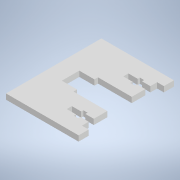
# Autodesk Inventor part: Soporte_Plug_Alimentacion
Saved by Autodesk Inventor 2020.1 (Build 241239000, 239)
## iProperties
Created: 2019-12-12
Part Number: Soporte_Plug_Alimentacion
Material: Generic
Document SubType Name: Modeling
Designer: Daniel
Density: 1 g/cm^3
Appearance: Default
Author: Daniel
Autodesk Inventor part; units mm, degrees
ref_plane "YZ Plane" through (0, 0, 0) normal (1, 0, 0) x (0, 1, 0)
ref_plane "XZ Plane" through (0, 0, 0) normal (0, 1, 0) x (-1, 0, 0)
ref_plane "XY Plane" through (0, 0, 0) normal (0, 0, 1) x (1, 0, 0)
sketch "Sketch1" plane through (0, 0, 0) normal (0, 1, 0) x (-1, 0, 0)
  line L0 (38.3151, 0) -> (38.3151, -28.25)
  line L1 (38.3151, -28.25) -> (-4.6849, -28.25)
  line L2 (-4.6849, -28.25) -> (-4.6849, -22.25)
  line L3 (-4.6849, -22.25) -> (-0.6849, -22.25)
  line L4 (-0.6849, -22.25) -> (-0.6849, -18.25)
  line L5 (-0.6849, -18.25) -> (4.3151, -18.25)
  line L6 (4.3151, -18.25) -> (4.3151, -19.525)
  line L7 (4.3151, -19.525) -> (6.8151, -19.525)
  line L8 (6.8151, -13.975) -> (4.3151, -13.975)
  line L9 (4.3151, -13.975) -> (4.3151, -15.25)
  line L10 (4.3151, -15.25) -> (-0.6849, -15.25)
  line L11 (-0.6849, -15.25) -> (-0.6849, -7.25)
  line L12 (-0.6849, -7.25) -> (19.3151, -7.25)
  line L13 (19.3151, -7.25) -> (19.3151, -5.15)
  line L14 (19.3151, -5.15) -> (28.3151, -5.15)
  line L15 (28.3151, -5.15) -> (28.3151, 0)
  line L16 (0, 0) -> (38.3151, 0) construction
  line L17 (6.8151, -15.25) -> (12.3151, -15.25)
  line L18 (12.3151, -15.25) -> (12.3151, -18.25)
  line L19 (12.3151, -18.25) -> (6.8151, -18.25)
  line L20 (6.8151, -19.525) -> (6.8151, -18.25)
  line L21 (6.8151, -15.25) -> (6.8151, -13.975)
  line L22 (38.3151, 0) -> (38.3151, 28.25)
  line L23 (38.3151, 28.25) -> (-4.6849, 28.25)
  line L24 (-4.6849, 28.25) -> (-4.6849, 22.25)
  line L25 (-4.6849, 22.25) -> (-0.6849, 22.25)
  line L26 (-0.6849, 22.25) -> (-0.6849, 18.25)
  line L27 (-0.6849, 18.25) -> (4.3151, 18.25)
  line L28 (4.3151, 18.25) -> (4.3151, 19.525)
  line L29 (4.3151, 19.525) -> (6.8151, 19.525)
  line L30 (6.8151, 13.975) -> (4.3151, 13.975)
  line L31 (4.3151, 13.975) -> (4.3151, 15.25)
  line L32 (4.3151, 15.25) -> (-0.6849, 15.25)
  line L33 (-0.6849, 15.25) -> (-0.6849, 7.25)
  line L34 (-0.6849, 7.25) -> (19.3151, 7.25)
  line L35 (19.3151, 7.25) -> (19.3151, 5.15)
  line L36 (19.3151, 5.15) -> (28.3151, 5.15)
  line L37 (28.3151, 5.15) -> (28.3151, 0)
  line L38 (6.8151, 15.25) -> (12.3151, 15.25)
  line L39 (12.3151, 15.25) -> (12.3151, 18.25)
  line L40 (12.3151, 18.25) -> (6.8151, 18.25)
  line L41 (6.8151, 19.525) -> (6.8151, 18.25)
  line L42 (6.8151, 15.25) -> (6.8151, 13.975)
  dimension "d0" = 5.55
  dimension "d1" = 2.5
  dimension "d2" = 3
  dimension "d3" = 6
  dimension "d4" = 5
  dimension "d7" = 4
  dimension "d9" = 24
  dimension "d10" = 17
  dimension "d11" = 10.3
  dimension "d12" = 9
  dimension "d13" = 14.5
  dimension "d14" = 8
  dimension "d15" = 4
  dimension "d16" = 10
  constraints: 86 end point, 20 symmetric about line, 18 perpendicular, 9 point on line, 4 collinear, 3 horizontal, 2 parallel, 1 other
  measures "d0" distance of L7.end L8.start
  measures "d1" distance of L6.end L7.end
  measures "d2" distance between parallel lines of L10 L5
  measures "d3" distance of L1.end L2.end
  measures "d4" distance of L4.end L5.end
  measures "d7" distance of L2.end L3.end
  measures "d9" distance between parallel lines of L2 L13
  measures "d10" distance between parallel lines of L2 L18
  measures "d11" diameter of L14 L16
  measures "d12" distance of L13.end L14.end
  measures "d13" diameter of L12 L16
  measures "d14" distance of L10.end L11.end
  measures "d15" distance of L3.end L4.end
  measures "d16" distance between parallel lines of L0 L15
extrude "Extrusion1" add sketch "Sketch1" along normal blind 3.2
body "Solid1"
